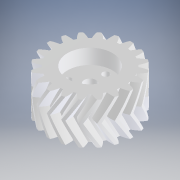
# Autodesk Inventor part: Spur Gear1
Saved by Autodesk Inventor 2017 SP1 (Build 210196100, 196)
## iProperties
Created: 2017-10-23
Part Number: Spur Gear1
Material: ABS Plastic
Document SubType Name: Modeling
Designer: Zach
Categories: <?xml version="1.0" encoding="UTF-16"?> <MemberInstance><Categories><FamilyTemplate><FamilyTemplateParameter ValueType="xs:double" Id="1" ObjectReferenceKey="da_z" ObjectType="kUserParameterObject"/><FamilyTemplateParameter ValueType="xs:double" Id="2" ObjectReferenceKey="da_b" ObjectType="kUserParameterObject"/><FamilyTemplateParameter ValueType="xs:double" Id="3" ObjectReferenceKey="da_beta" ObjectType="kUserParameterObject"/><FamilyTemplateParameter ValueType="xs:double" Id="4" ObjectReferenceKey="da_da" ObjectType="kUserParameterObject"/><FamilyTemplateParameter ValueType="xs:double" Id="5" ObjectReferenceKey="da_aw" ObjectType="kUserParameterObject"/><FamilyTemplateParameter ValueType="xs:string" Id="6" ObjectReferenceKey="EAIAABAAAACIAQAAAAAAAIAAAAAAAAAA" ObjectType="83910656" SubObjectId="SurfaceGeometry"/></FamilyTemplate><ParamToTemplateMap><ParamToTemplate CategoryParameter="//CategoryParameter[@InternalName='046C89C9-8512-4d59-83FE-43B91F4F132A']" TemplateParameter="1"/><ParamToTemplate CategoryParameter="//CategoryParameter[@InternalName='2552DF32-E462-4b46-AEBF-C6C7768E72AC']" TemplateParameter="2"/><ParamToTemplate CategoryParameter="//CategoryParameter[@InternalName='C9EE641D-15FC-4fae-A226-E94C4372FDD7']" TemplateParameter="3"/><ParamToTemplate><ParamToTemplate CategoryParameter="//CategoryParameter[@InternalName='00B6519A-459B-49c7-AD84-2E56D39A5744']" ConstantValue="0.000000"/></ParamToTemplate><ParamToTemplate><ParamToTemplate CategoryParameter="//CategoryParameter[@InternalName='04B31F0E-C7A6-4894-AA32-9629BEFACF47']" ConstantValue="1.000000"/></ParamToTemplate><ParamToTemplate><ParamToTemplate CategoryParameter="//CategoryParameter[@InternalName='43CBEC2E-7847-49e7-A936-2F7889FCB2D9']" ConstantValue="0.250000"/></ParamToTemplate><ParamToTemplate><ParamToTemplate CategoryParameter="//CategoryParameter[@InternalName='B1EFC894-105D-4ebd-86BF-FA20ED196853']" ConstantValue="0.350000"/></ParamToTemplate><ParamToTemplate><ParamToTemplate CategoryParameter="//CategoryParameter[@InternalName='51175063-3D10-4879-93E8-6246FE8B403D']" ConstantValue="2060000000.000000"/></ParamToTemplate><ParamToTemplate><ParamToTemplate CategoryParameter="//CategoryParameter[@InternalName='A3A52E27-4454-46a9-B0BD-C932399B70AF']" ConstantValue="0.300000"/></ParamToTemplate><ParamToTemplate><ParamToTemplate CategoryParameter="//CategoryParameter[@InternalName='91B76062-C214-41d9-B1B9-14D2AB99603D']" ConstantValue="0.200000"/></ParamToTemplate><ParamToTemplate><ParamToTemplate CategoryParameter="//CategoryParameter[@InternalName='374E806E-8B8A-4dda-A9AA-1039D6500AD2']" ConstantValue="5.000000"/></ParamToTemplate><ParamToTemplate><ParamToTemplate CategoryParameter="//CategoryParameter[@InternalName='2D373A89-B862-43d6-8D0B-0CBF12AB9F6C']" ConstantValue="0.392699"/></ParamToTemplate><ParamToTemplate CategoryParameter="//CategoryParameter[@InternalName='37777632-D6A2-4fac-9D53-DB8ACD95C989']" TemplateParameter="4"/><ParamToTemplate CategoryParameter="//CategoryParameter[@InternalName='FD1017F1-B727-4f7e-9707-0F86F1FF9423']" TemplateParameter="5"/><ParamToTemplate><ParamToTemplate CategoryParameter="//CategoryParameter[@InternalName='9E1B4470-B2D3-4ff1-B813-535BB4CDF51A']" ConstantValue="3520000.000000"/></ParamToTemplate><ParamToTemplate><ParamToTemplate CategoryParameter="//CategoryParameter[@InternalName='F8452263-BFF6-458c-9FB1-07C4B99E95CD']" ConstantValue="11400000.000000"/></ParamToTemplate><ParamToTemplate><ParamToTemplate CategoryParameter="//CategoryParameter[@InternalName='3E3BB259-FD49-497f-8171-6EBC954A3479']" ConstantValue="2.000000"/></ParamToTemplate><ParamToTemplate CategoryParameter="//CategoryParameter[@InternalName='27C3BAF2-7550-4e4b-AE2C-0DB134B7D9B7']" TemplateParameter="6"/></ParamToTemplateMap><Category DisplayName="Gear" InternalName="DC85795E-93AB-48d5-8EEE-5A27447B64BD" Mnemonic="Gear"><CategoryParameter DisplayName="z" InternalName="046C89C9-8512-4d59-83FE-43B91F4F132A" Mnemonic="z"/><CategoryParameter DisplayName="b" InternalName="2552DF32-E462-4b46-AEBF-C6C7768E72AC" Mnemonic="b"/><CategoryParameter DisplayName="||b|" InternalName="C9EE641D-15FC-4fae-A226-E94C4372FDD7" Mnemonic="beta"/><CategoryParameter DisplayName="x" InternalName="00B6519A-459B-49c7-AD84-2E56D39A5744" Mnemonic="x"/><CategoryParameter DisplayName="a*" InternalName="04B31F0E-C7A6-4894-AA32-9629BEFACF47" Mnemonic="a"/><CategoryParameter DisplayName="c*" InternalName="43CBEC2E-7847-49e7-A936-2F7889FCB2D9" Mnemonic="c"/><CategoryParameter DisplayName="r|.f|*" InternalName="B1EFC894-105D-4ebd-86BF-FA20ED196853" Mnemonic="rf"/><CategoryParameter DisplayName="E" InternalName="51175063-3D10-4879-93E8-6246FE8B403D" Mnemonic="E"/><CategoryParameter DisplayName="||m|" InternalName="A3A52E27-4454-46a9-B0BD-C932399B70AF" Mnemonic="mi"/><Category DisplayName="SpurGear" InternalName="26C5A22E-A91E-4dfd-A3B3-23CCAFAE1764" Mnemonic="SpurGear"><CategoryParameter DisplayName="m" InternalName="91B76062-C214-41d9-B1B9-14D2AB99603D" Mnemonic="m"/><CategoryParameter DisplayName="P" InternalName="374E806E-8B8A-4dda-A9AA-1039D6500AD2" Mnemonic="PP"/><CategoryParameter DisplayName="||a|" InternalName="2D373A89-B862-43d6-8D0B-0CBF12AB9F6C" Mnemonic="alpha"/><CategoryParameter DisplayName="d|.a|" InternalName="37777632-D6A2-4fac-9D53-DB8ACD95C989" Mnemonic="da"/><CategoryParameter DisplayName="a|.w|" InternalName="FD1017F1-B727-4f7e-9707-0F86F1FF9423" Mnemonic="aw"/><CategoryParameter DisplayName="||s||.Flim|" InternalName="9E1B4470-B2D3-4ff1-B813-535BB4CDF51A" Mnemonic="sFlim"/><CategoryParameter DisplayName="||s||.Hlim|" InternalName="F8452263-BFF6-458c-9FB1-07C4B99E95CD" Mnemonic="sHlim"/><CategoryParameter DisplayName="type" InternalName="3E3BB259-FD49-497f-8171-6EBC954A3479" Mnemonic="type"/><CategoryParameter DisplayName="PitchDiameter" InternalName="27C3BAF2-7550-4e4b-AE2C-0DB134B7D9B7" Mnemonic="IDS_PITCHDIAM"/></Category></Category></Categories></MemberInstance>
Density: 1.06 g/cm^3
Appearance: CR White
CustomPartVersion: 1
Author: Zach
Autodesk Inventor part; units mm, degrees
sketch "Sketch1" plane through (0, 0, 0) normal (0, 0, 1) x (1, 0, 0)
  circle A0 centre (0, 0) radius 25.0821
  dimension "d0" = 50.1642
  constraints: 1 centre point
  measures "d0" diameter of A0
extrude "Extrusion1" add sketch "Sketch1" along normal blind 12.5
ref_plane "Work Plane2" through (0, 0, 6.25) normal (0, 0, 1) x (1, 0, 0)
sketch "Sketch2" plane through (0, 0, 0) normal (0, 0, -1) x (-1, 0, 0)
  circle A0 centre (0, 0) radius 25.0821 projected
  circle A1 centre (0, 0) radius 23.2857
  dimension "d3" = 46.5714
  constraints: 1 centre point, 1 coincident
  measures "d3" diameter of A1
surface extrude "Pitch Diameter" sketch "Sketch2" against normal through all shown no curves A1
ref_plane "Work Plane8" through (0, 0, 0) normal (0.9876883, 0.1564345, 0) x (0, 0, 1)
ref_plane "Work Plane9" through (0, 0, 0) normal (1, 0, 0) x (0, 1, 0)
spur gear teeth "Spur Gear" teeth 20 pitch diameter 46.188 tip diameter 50.1642 root diameter 41.188 face width 12.5 helix angle 30 hand left start plane through (0, 0, 0) normal (0, 0, -1) x (-1, 0, 0)
mirror "Mirror1" about plane through (0, 0, 12.5) normal (0, 0, 1)
sketch "Sketch3" plane through (-14.8399, 17.3808, 25) normal (0, 0, 1) x (0.9845988, 0.1748292, 0)
  circle A0 centre (11.5726, -19.7076) radius 13.5
  arc A1 (1.4985, 3.2624) -> (-0.2727, 2.4012) centre (11.5726, -19.7076) ccw construction
  arc A2 (-5.1066, -0.9749) -> (-6.5249, -2.3413) centre (11.5726, -19.7076) ccw construction
  arc A3 (-10.079, -7.0459) -> (-11.0057, -8.7837) centre (11.5726, -19.7076) ccw construction
  arc A4 (-12.932, -14.3563) -> (-13.2763, -16.2954) centre (11.5726, -19.7076) ccw construction
  arc A5 (-13.3862, -22.1906) -> (-13.1145, -24.1412) centre (11.5726, -19.7076) ccw construction
  arc A6 (-11.3974, -29.7818) -> (-10.5362, -31.5529) centre (11.5726, -19.7076) ccw construction
  arc A7 (-7.1601, -36.3868) -> (-5.7937, -37.8052) centre (11.5726, -19.7076) ccw construction
  arc A8 (-1.089, -41.3592) -> (0.6488, -42.2859) centre (11.5726, -19.7076) ccw construction
  arc A9 (6.2214, -44.2122) -> (8.1605, -44.5565) centre (11.5726, -19.7076) ccw construction
  arc A10 (14.0556, -44.6665) -> (16.0062, -44.3947) centre (11.5726, -19.7076) ccw construction
  arc A11 (21.6468, -42.6776) -> (23.418, -41.8164) centre (11.5726, -19.7076) ccw construction
  arc A12 (28.2519, -38.4403) -> (29.6702, -37.0739) centre (11.5726, -19.7076) ccw construction
  arc A13 (33.2243, -32.3693) -> (34.1509, -30.6315) centre (11.5726, -19.7076) ccw construction
  arc A14 (36.0772, -25.0588) -> (36.4215, -23.1197) centre (11.5726, -19.7076) ccw construction
  arc A15 (36.5315, -17.2246) -> (36.2598, -15.274) centre (11.5726, -19.7076) ccw construction
  arc A16 (34.5426, -9.6334) -> (33.6814, -7.8623) centre (11.5726, -19.7076) ccw construction
  arc A17 (30.3053, -3.0284) -> (28.9389, -1.61) centre (11.5726, -19.7076) ccw construction
  arc A18 (24.2343, 1.944) -> (22.4965, 2.8707) centre (11.5726, -19.7076) ccw construction
  arc A19 (16.9239, 4.797) -> (14.9848, 5.1413) centre (11.5726, -19.7076) ccw construction
  arc A20 (9.0896, 5.2513) -> (7.139, 4.9795) centre (11.5726, -19.7076) ccw construction
  dimension "d49" = 27
  constraints: 2 coincident, 1 centre point, 60 other
  measures "d49" diameter of A0
extrude "Extrusion2" cut sketch "Sketch3" against normal blind 9
sketch "Sketch4" plane through (0, 0, 16) normal (0, 0, 1) x (1, 0, 0)
  circle A0 centre (0, 0) radius 3.5
  circle A1 centre (0, 9.525) radius 2
  circle A2 centre (-8.2489, -4.7625) radius 2
  circle A3 centre (8.2489, -4.7625) radius 2
  circle A4 centre (0, 0) radius 13.5 construction
  dimension "d52" = 7
  dimension "d53" = 4
  dimension "d54" = 9.525
  dimension "d57" = 360
  constraints: 4 centre point, 1 coincident, 1 vertical alignment, 7 other
  measures "d52" diameter of A0
  measures "d53" diameter of A1
  measures "d54" distance of A1.centre point (0, 0)
extrude "Extrusion3" cut sketch "Sketch4" against normal through all
sketch "Sketch5" plane through (0, 0, 0) normal (0, 0, -1) x (-1, 0, 0)
  circle A0 centre (-8.2489, -4.7625) radius 2 projected
  circle A1 centre (-8.2489, -4.7625) radius 3.5
  circle A2 centre (8.2489, -4.7625) radius 3.5
  circle A3 centre (0, 9.525) radius 3.5
  point P0 (0, 0)
  dimension "d61" = 7
  dimension "d64" = 360
  constraints: 3 centre point, 1 coincident, 7 other
  measures "d61" diameter of A1
extrude "Extrusion4" cut sketch "Sketch5" against normal blind 11 contours A0 | A1 | A2 | A3
equation "\"d0\" = da_da"
equation "\"d1\" = da_b"
equation "\"d3\" = da_dw"
equation "\"d16\" = da_aw"
equation "\"d43\" = da_aw"
equation "\"d46\" = da_aw"
equation "\"da_da\" = 50.164157"
equation "\"da_b\" = 12.5"
equation "\"da_dw\" = 46.571429"
equation "\"da_aw\" = 81.5"
body "Solid1"
body "Srf1"
